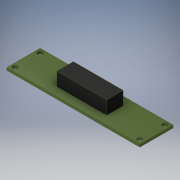
# Autodesk Inventor part: КВ33.044.1003 - Плата контроля сервомоторами
Saved by Autodesk Inventor 2019 (Build 230136000, 136)
## iProperties
Created: 2019-10-30
Part Number: КВ33.044.1003 - Плата контроля сервомоторами
Material: Серебро
Document SubType Name: Modeling
Designer: Петров Иван
Density: 10.49 g/cm^3
Appearance: Темно-оливковый
Author: Петров Иван
Autodesk Inventor part; units mm, degrees
ref_plane "YZ Plane" through (0, 0, 0) normal (1, 0, 0) x (0, 1, 0)
ref_plane "XZ Plane" through (0, 0, 0) normal (0, 1, 0) x (-1, 0, 0)
ref_plane "XY Plane" through (0, 0, 0) normal (0, 0, 1) x (1, 0, 0)
sketch "Эскиз1" plane through (0, 0, 0) normal (0, 1, 0) x (-1, 0, 0)
  line L0 (-40, 10) -> (40, 10)
  line L1 (40, 10) -> (40, -10)
  line L2 (40, -10) -> (-40, -10)
  line L3 (-40, -10) -> (-40, 10)
  line L4 (-40, 10) -> (40, -10) construction
  line L5 (40, 10) -> (-40, -10) construction
  point P0 (0, 0)
  dimension "d0" = 80
  dimension "d1" = 20
  constraints: 12 end point, 2 midpoint, 2 parallel, 1 horizontal, 1 perpendicular
  measures "d0" distance of L1.end L2.end
  measures "d1" distance of L0.end L1.end
extrude "Выдавливание1" add sketch "Эскиз1" along normal blind 1.6
sketch "Эскиз2" plane through (0, 1.6, 0) normal (0, 1, 0) x (1, 0, 0)
  line L0 (-37.5, -7.5) -> (-37.5, 7.5)
  line L1 (37.5, 7.5) -> (37.5, -7.5)
  circle A0 centre (-37.5, -7.5) radius 1.5
  circle A1 centre (-37.5, 7.5) radius 1.5
  circle A2 centre (37.5, 7.5) radius 1.5
  circle A3 centre (37.5, -7.5) radius 1.5
  point P0 (0, 0)
  dimension "d4" = 75
  dimension "d5" = 15
  dimension "d6" = 3
  dimension "d7" = 3
  dimension "d8" = 3
  dimension "d9" = 3
  constraints: 4 centre point, 4 coincident, 4 end point, 1 parallel
  measures "d4" distance of L0.end L1.start
  measures "d5" distance of L0.start L0.end
  measures "d6" diameter of A0
  measures "d7" diameter of A1
  measures "d8" diameter of A2
  measures "d9" diameter of A3
extrude "Выдавливание2" cut sketch "Эскиз2" against normal blind 1.6
sketch "Эскиз3" plane through (0, 1.6, 0) normal (0, 1, 0) x (1, 0, 0)
  line L0 (15, -5) -> (-15, -5)
  line L1 (-15, -5) -> (-15, 5)
  line L2 (-15, 5) -> (15, 5)
  line L3 (15, 5) -> (15, -5)
  line L4 (15, -5) -> (-15, 5) construction
  line L5 (-15, -5) -> (15, 5) construction
  point P0 (0, 0)
  dimension "d12" = 30
  dimension "d13" = 10
  constraints: 12 end point, 2 midpoint, 2 parallel, 1 horizontal, 1 perpendicular
  measures "d12" distance of L1.end L2.end
  measures "d13" distance of L0.end L1.end
extrude "Выдавливание3" add sketch "Эскиз3" along normal blind 8
